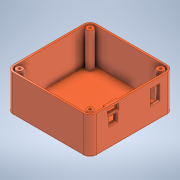
# Autodesk Inventor part: Arduino_case_bottom_JC_Rev2
Saved by Autodesk Inventor 2020 (Build 240168000, 168)
## iProperties
Created: 2019-08-28
Part Number: Arduino_case_bottom_JC_Rev2
Material: Generic
Document SubType Name: Modeling
Designer: jcocker
Density: 1 g/cm^3
Appearance: Smooth - Light Orange
Author: jcocker
Autodesk Inventor part; units mm, degrees
ref_plane "YZ Plane" through (0, 0, 0) normal (1, 0, 0) x (0, 1, 0)
ref_plane "XZ Plane" through (0, 0, 0) normal (0, 1, 0) x (-1, 0, 0)
ref_plane "XY Plane" through (0, 0, 0) normal (0, 0, 1) x (1, 0, 0)
sketch "Sketch1" plane through (0, 0, 0) normal (0, 1, 0) x (-1, 0, 0)
  line L0 (-33.65, -40) -> (33.65, -40)
  line L1 (40, -33.65) -> (40, 33.65)
  line L2 (33.65, 40) -> (-33.65, 40)
  line L3 (-40, 33.65) -> (-40, -33.65)
  line L4 (-40, -40) -> (40, 40) construction
  line L5 (40, -40) -> (-40, 40) construction
  arc A0 (40, 33.65) -> (33.65, 40) centre (33.65, 33.65) ccw
  arc A1 (-33.65, 40) -> (-40, 33.65) centre (-33.65, 33.65) ccw
  arc A2 (-40, -33.65) -> (-33.65, -40) centre (-33.65, -33.65) ccw
  arc A3 (33.65, -40) -> (40, -33.65) centre (33.65, -33.65) ccw
  point P0 (0, 0)
  dimension "d0" = 80
  dimension "d1" = 80
  dimension "d2" = 6.35
  constraints: 12 end point, 8 point on circle, 8 point on line, 8 tangent, 4 centre point, 3 equal radius, 2 midpoint, 2 parallel, 1 horizontal, 1 perpendicular
  measures "d0" distance of L5.end L4.end
  measures "d1" distance of L4.end L5.start
  measures "d2" radius of A0
extrude "Extrusion1" add sketch "Sketch1" along normal blind 25.4
shell "Shell1" thickness 1.7 removed faces 1 at (-11.2167, 25.4, 9.1)
fillet "Fillet1" radius 1.27 8 edges at (-38.1401, 0, -38.1401) (-40, 0, 0) (-38.1401, 0, 38.1401) (0, 0, 40) (38.1401, 0, 38.1401) (40, 0, 0) (38.1401, 0, -38.1401) (0, 0, -40)
sketch "Sketch2" plane through (-33.65, 1.7, 38.3) normal (0, 1, 0) x (1, 0, 0)
  arc A0 (-4.65, 4.65) -> (0, 0) centre (0, 4.65) ccw projected
  circle A1 centre (0, 4.65) radius 3.175
  circle A2 centre (0, 4.65) radius 1.2
  point P0 (33.65, 38.3)
  dimension "d7" = 6.35
  dimension "d8" = 2.4
  constraints: 2 centre point, 2 coincident
  measures "d7" diameter of A1
  measures "d8" diameter of A2
extrude "Extrusion2" add sketch "Sketch2" along normal up to surface (23.7 mm away)
mirror "Mirror1" about plane through (0, 0, 0) normal (1, 0, 0) of "Extrusion2"
mirror "Mirror2" about plane through (0, 0, 0) normal (0, 0, 1) of "Extrusion2", "Mirror1"
sketch "Sketch4" plane through (0, 25.4, 0) normal (0, 1, 0) x (1, 0, 0)
  line L0 (-38.3, -33.65) -> (-38.3, 33.65) projected
  arc A0 (-33.65, 38.3) -> (-38.3, 33.65) centre (-33.65, 33.65) ccw projected
  line L1 (-33.65, 38.3) -> (33.65, 38.3) projected
  arc A1 (38.3, 33.65) -> (33.65, 38.3) centre (33.65, 33.65) ccw projected
  line L2 (38.3, 33.65) -> (38.3, -33.65) projected
  arc A2 (33.65, -38.3) -> (38.3, -33.65) centre (33.65, -33.65) ccw projected
  line L3 (33.65, -38.3) -> (-33.65, -38.3) projected
  arc A3 (-38.3, -33.65) -> (-33.65, -38.3) centre (-33.65, -33.65) ccw projected
  arc A4 (-40, -33.65) -> (-33.65, -40) centre (-33.65, -33.65) ccw projected
  line L4 (-33.65, -40) -> (33.65, -40) projected
  arc A5 (33.65, -40) -> (40, -33.65) centre (33.65, -33.65) ccw projected
  line L5 (40, -33.65) -> (40, 33.65) projected
  arc A6 (40, 33.65) -> (33.65, 40) centre (33.65, 33.65) ccw projected
  line L6 (33.65, 40) -> (-33.65, 40) projected
  arc A7 (-33.65, 40) -> (-40, 33.65) centre (-33.65, 33.65) ccw projected
  line L7 (-40, 33.65) -> (-40, -33.65) projected
  circle A8 centre (-33.65, 33.65) radius 1.2 projected
  circle A9 centre (-33.65, 33.65) radius 3.175 projected
  circle A10 centre (-33.65, -33.65) radius 1.2 projected
  circle A11 centre (-33.65, -33.65) radius 3.175 projected
  circle A12 centre (33.65, -33.65) radius 1.2 projected
  circle A13 centre (33.65, -33.65) radius 3.175 projected
  circle A14 centre (33.65, 33.65) radius 1.2 projected
  circle A15 centre (33.65, 33.65) radius 3.175 projected
  point P0 (0, 0)
extrude "Extrusion4" add sketch "Sketch4" along normal blind 10
sketch "Sketch5" plane through (-33.65, 1.7, 38.3) normal (0, 1, 0) x (1, 0, 0)
  line L0 (71.95, 71.95) -> (71.95, 4.65) projected
  line L1 (71.95, 13.9457) -> (70.68, 13.9457)
  line L2 (70.68, 13.9457) -> (70.68, 26.6457)
  line L3 (70.68, 26.6457) -> (71.95, 26.6457)
  line L4 (71.95, 26.6457) -> (71.95, 13.9457)
  point P0 (33.65, 38.3)
  dimension "d18" = 1.27
  dimension "d19" = 12.7
  constraints: 8 end point, 2 parallel, 1 horizontal, 1 perpendicular, 1 point on line
  measures "d18" distance of L2.end L3.end
  measures "d19" distance of L1.end L2.end
extrude "Extrusion5" add sketch "Sketch5" along normal up to surface (33.7 mm away)
sketch "Sketch6" plane through (37.03, 1.7, 11.6543) normal (-1, 0, 0) x (0, 0, 1)
  line L0 (10.75, 30.7) -> (1.75, 30.7)
  line L1 (1.75, 30.7) -> (1.75, 26.7)
  line L2 (1.75, 26.7) -> (10.75, 26.7)
  line L3 (10.75, 26.7) -> (10.75, 30.7)
  line L4 (0, 0) -> (0, 33.7) projected
  line L5 (21.9957, 33.7) -> (-45.3043, 33.7) projected
  line L6 (3.05, 17.3) -> (9.45, 17.3)
  line L7 (9.45, 17.3) -> (9.45, 23.7)
  line L8 (9.45, 23.7) -> (3.05, 23.7)
  line L9 (3.05, 23.7) -> (3.05, 17.3)
  line L10 (3.05, 17.3) -> (9.45, 23.7) construction
  line L11 (9.45, 17.3) -> (3.05, 23.7) construction
  point P0 (-11.6543, -1.7)
  point P1 (6.25, 20.5)
  dimension "d22" = 9
  dimension "d23" = 4
  dimension "d24" = 1.75
  dimension "d25" = 3
  dimension "d26" = 6.4
  dimension "d27" = 6.4
  dimension "d28" = 3
  constraints: 20 end point, 4 parallel, 2 horizontal, 2 midpoint, 2 perpendicular
  measures "d22" distance of L2.end L1.end
  measures "d23" distance of L1.end L0.end
  measures "d24" distance between parallel lines of L4 L1
  measures "d25" distance between parallel lines of L5 L0
  measures "d26" distance of L8.end L7.end
  measures "d27" distance of L7.end L6.end
  measures "d28" distance between parallel lines of L2 L8
extrude "Extrusion6" cut sketch "Sketch6" against normal blind 10
chamfer "Chamfer1" distance 1 angle 45 8 edges at (40, 28.4, 17.9043) (40, 30.4, 22.4043) (40, 32.4, 17.9043) (40, 30.4, 13.4043) (40, 22.2, 21.1043) (40, 22.2, 14.7043) (40, 19, 17.9043) (40, 25.4, 17.9043)
sketch "Sketch7" plane through (40, 1.27, 33.65) normal (1, 0, 0) x (0, 0, -1)
  line L0 (59.68, 14.826) -> (51.806, 14.826)
  line L1 (51.806, 14.826) -> (51.806, 27.78)
  line L2 (51.806, 27.78) -> (59.68, 27.78)
  line L3 (59.68, 27.78) -> (59.68, 14.826)
  line L4 (59.68, 14.826) -> (51.806, 27.78) construction
  line L5 (51.806, 14.826) -> (59.68, 27.78) construction
  line L6 (0, 34.13) -> (67.3, 34.13) projected
  line L7 (67.3, 0) -> (67.3, 34.13) projected
  point P0 (33.65, -1.27)
  point P1 (55.743, 21.303)
  dimension "d34" = 7.874
  dimension "d35" = 12.954
  dimension "d36" = 6.35
  dimension "d37" = 7.62
  constraints: 12 end point, 2 midpoint, 2 parallel, 1 horizontal, 1 perpendicular
  measures "d34" distance of L1.end L2.end
  measures "d35" distance of L0.end L1.end
  measures "d36" distance between parallel lines of L6 L2
  measures "d37" distance between parallel lines of L7 L3
extrude "Extrusion7" cut sketch "Sketch7" against normal blind 25.4
chamfer "Chamfer2" distance 0.762 angle 45 4 edges at (40, 22.573, -18.156) (40, 16.096, -22.093) (40, 29.05, -22.093) (40, 22.573, -26.03)
body "Solid1"
